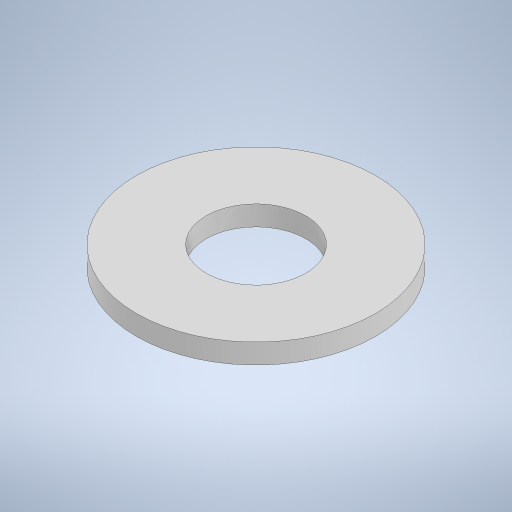
# Autodesk Inventor part: Rondella
Saved by Autodesk Inventor 2023 (Build 270158000, 158)
## iProperties
Created: 2026-01-13
Part Number: Rondella
Material: Generico
Document SubType Name: Modeling
Designer: Davide
Density: 1 g/cm^3
Appearance: Default
1_Materiale: − − −
2_Trattamento: − − −
3_Disegnato: D. Mitidieri
4_Controllato: C. Pirrottina
5_Approvato: S. Musella
Author: Davide
Autodesk Inventor part; units mm, degrees
ref_plane "YZ Plane" through (0, 0, 0) normal (1, 0, 0) x (0, 1, 0)
ref_plane "XZ Plane" through (0, 0, 0) normal (0, 1, 0) x (-1, 0, 0)
ref_plane "XY Plane" through (0, 0, 0) normal (0, 0, 1) x (1, 0, 0)
sketch "Schizzo1" plane through (0, 0, 0) normal (0, 1, 0) x (-1, 0, 0)
  circle A0 centre (0, 0) radius 3
  circle A1 centre (0, 0) radius 1.25
  dimension "d0" = 6
  dimension "d1" = 2.5
  constraints: 2 centre point, 2 coincident
  measures "d0" diameter of A0
  measures "d1" diameter of A1
extrude "Estrusione1" add sketch "Schizzo1" along normal mid plane 0.5
equation "\"d0\" = od"
equation "\"d1\" = d"
equation "\"d2\" = spess"
equation "\"d\" = 2.5"
equation "\"od\" = 6"
equation "\"spess\" = 0.5"
